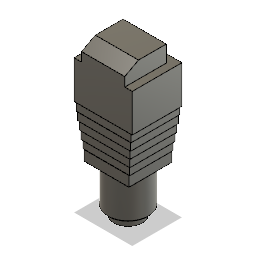
DIYbio orbital shaker bottom case (Autodesk Fusion 360 archive; units mm, degrees)
design "greenPlug"
Autodesk Fusion 360 part; units mm, degrees
sketch "Sketch1" plane through (0, 0, 0) normal (0, 1, 0) x (1, 0, 0)
  line L0 (5.245, -3.385) -> (-5.245, -3.385)
  line L1 (-5.245, -3.385) -> (-5.245, 3.385)
  line L2 (-5.245, 3.385) -> (5.245, 3.385)
  line L3 (5.245, 3.385) -> (5.245, -3.385)
  line L4 (5.245, -3.385) -> (-5.245, 3.385) construction
  line L5 (-5.245, -3.385) -> (5.245, 3.385) construction
  line L6 (5.245, -6.6889) -> (-5.245, -6.6889)
  line L7 (-5.245, -6.6889) -> (-5.245, -3.3689)
  line L8 (-5.245, -3.3689) -> (5.245, -3.3689)
  line L9 (5.245, -3.3689) -> (5.245, -6.6889)
  line L10 (5.245, -6.6889) -> (-5.245, -3.3689) construction
  line L11 (-5.245, -6.6889) -> (5.245, -3.3689) construction
  point P0 (0, -5.0289)
  dimension "d1" = 6.77
  dimension "d2" = 10.49
  dimension "d5" = 3.32
  dimension "d6" = 10.49
  constraint perpendicular L0 L1
  constraint parallel L0 L2
  constraint parallel L1 L3
  constraint horizontal L0
  constraint coincident L4 origin
  constraint coincident L5 origin
  constraint perpendicular L6 L7
  constraint parallel L6 L8
  constraint parallel L7 L9
  constraint horizontal L6
  constraint coincident L10 P0
  constraint coincident L11 P0
  measures "d1" distance of L0.end L1.end
  measures "d2" distance of L1.end L2.end
  measures "d5" distance of L6.end L7.end
  measures "d6" distance of L7.end L8.end
extrude "Extrude2" add sketch "Sketch1" along normal blind 3.99 contours L0 L6 L7 L9
extrude "Extrude1" add sketch "Sketch1" along normal blind 3.99 contours L0 L1 L3 L7 L8 L9 | L1 L2 L3 L8
sketch "Sketch2" plane through (-5.245, 0, 0) normal (-1, 0, 0) x (0, 0, 1)
  line L0 (-3.385, 0) -> (6.6889, 0)
  line L1 (6.6889, 0) -> (6.6889, 3.99)
  line L2 (6.6889, 3.99) -> (-3.385, 3.99)
  line L3 (-3.385, 3.99) -> (-3.385, 0)
  line L4 (6.6889, 3.99) -> (6.6889, 2.2)
  line L5 (6.6889, 3.99) -> (3.3689, 3.99)
  line L6 (3.3689, 3.99) -> (6.6889, 2.2)
  dimension "d9" = 1.79
  dimension "d10" = 3.32
  constraint coincident L1.end L2.start
  constraint perpendicular L2 L4
  constraint perpendicular L1 L5
  measures "d9" distance of L1.end L4.end
  measures "d10" distance of L1.end L5.end
extrude "Extrude3" cut sketch "Sketch2" against normal up to surface (10.49 mm away) contours L1 L2 L4 L5 L6
sketch "Sketch4" plane through (0, 0, 0) normal (0, -1, 0) x (1, 0, 0)
  line L0 (5.245, -3.385) -> (5.245, 6.6889)
  line L1 (5.245, 6.6889) -> (-5.245, 6.6889)
  line L2 (-5.245, 6.6889) -> (-5.245, -3.385)
  line L3 (-5.245, -3.385) -> (5.245, -3.385)
  line L4 (-7.055, 6.6889) -> (7.055, 6.6889)
  line L5 (7.055, 6.6889) -> (7.055, -5.3611)
  line L6 (7.055, -5.3611) -> (-7.055, -5.3611)
  line L7 (-7.055, -5.3611) -> (-7.055, 6.6889)
  line L8 (5.245, 3.3689) -> (5.245, 6.6889)
  dimension "d15" = 14.11
  dimension "d16" = 12.05
  dimension "d19" = 1.81
  constraint horizontal L4
  constraint vertical L5
  constraint horizontal L6
  constraint vertical L7
  measures "d15" distance of L4.start L4.end
  measures "d16" distance of L4.start L6.end
  measures "d19" distance of L5 L8
extrude "Extrude4" add sketch "Sketch4" 1 faces at (-1.7483, 0, -0.027) along normal blind 9.14 contours L0 L2 L3 L4 L5 L6 L7 L8
sketch "Sketch5" plane through (0, -9.14, 0) normal (0, -1, 0) x (1, 0, 0)
  line L0 (-7.055, -5.3611) -> (7.055, -5.3611)
  line L1 (7.055, -5.3611) -> (7.055, 6.6889)
  line L2 (7.055, 6.6889) -> (-7.055, 6.6889)
  line L3 (-7.055, 6.6889) -> (-7.055, -5.3611)
  line L4 (-6.61, 6.5539) -> (6.61, 6.5539)
  line L5 (6.61, 6.5539) -> (6.61, -5.2261)
  line L6 (6.61, -5.2261) -> (-6.61, -5.2261)
  line L7 (-6.61, -5.2261) -> (-6.61, 6.5539)
  dimension "d20" = 13.22
  dimension "d21" = 11.78
  dimension "d24" = 0.445
  dimension "d25" = 0.135
  constraint horizontal L4
  constraint vertical L5
  constraint horizontal L6
  constraint vertical L7
  measures "d20" distance of L4.start L4.end
  measures "d21" distance of L4.start L6.end
  measures "d24" distance of L3 L7
  measures "d25" distance of L2 L4
extrude "Extrude5" add sketch "Sketch5" along normal blind 1.92 contours L4 L5 L6 L7
sketch "Sketch6" plane through (0, -11.06, 0) normal (0, -1, 0) x (1, 0, 0)
  line L0 (-6.61, -5.2261) -> (6.61, -5.2261)
  line L1 (6.61, -5.2261) -> (6.61, 6.5539)
  line L2 (6.61, 6.5539) -> (-6.61, 6.5539)
  line L3 (-6.61, 6.5539) -> (-6.61, -5.2261)
  line L4 (6.415, -5.1311) -> (-6.415, -5.1311)
  line L5 (-6.415, -5.1311) -> (-6.415, 6.4589)
  line L6 (-6.415, 6.4589) -> (6.415, 6.4589)
  line L7 (6.415, 6.4589) -> (6.415, -5.1311)
  line L8 (6.415, -5.1311) -> (-6.415, 6.4589) construction
  line L9 (-6.415, -5.1311) -> (6.415, 6.4589) construction
  point P0 (0, 0.6639)
  dimension "d26" = 12.83
  dimension "d27" = 11.59
  dimension "d28" = 0.195
  dimension "d29" = 0.095
  constraint perpendicular L4 L5
  constraint parallel L4 L6
  constraint parallel L5 L7
  constraint horizontal L4
  constraint coincident L8 P0
  constraint coincident L9 P0
  measures "d26" distance of L5.end L6.end
  measures "d27" distance of L4.end L5.end
  measures "d28" distance of L1 L7
  measures "d29" distance of L0 L4
extrude "Extrude6" add sketch "Sketch6" along normal blind 1.92 contours L4 L5 L6 L7
sketch "Sketch7" plane through (0, -12.98, 0) normal (0, -1, 0) x (1, 0, 0)
  line L0 (6.415, 6.4589) -> (-6.415, 6.4589)
  line L1 (-6.415, 6.4589) -> (-6.415, -5.1311)
  line L2 (-6.415, -5.1311) -> (6.415, -5.1311)
  line L3 (6.415, -5.1311) -> (6.415, 6.4589)
  line L4 (6.12, -4.9711) -> (-6.12, -4.9711)
  line L5 (-6.12, -4.9711) -> (-6.12, 6.2989)
  line L6 (-6.12, 6.2989) -> (6.12, 6.2989)
  line L7 (6.12, 6.2989) -> (6.12, -4.9711)
  line L8 (6.12, -4.9711) -> (-6.12, 6.2989) construction
  line L9 (-6.12, -4.9711) -> (6.12, 6.2989) construction
  point P0 (0, 0.6639)
  dimension "d32" = 12.24
  dimension "d33" = 11.27
  dimension "d34" = 0.16
  dimension "d35" = 0.295
  constraint perpendicular L4 L5
  constraint parallel L4 L6
  constraint parallel L5 L7
  constraint horizontal L4
  constraint coincident L8 P0
  constraint coincident L9 P0
  measures "d32" distance of L5.end L6.end
  measures "d33" distance of L4.end L5.end
  measures "d34" distance of L2 L4
  measures "d35" distance of L3 L7
extrude "Extrude7" add sketch "Sketch7" along normal blind 1.92 contours L4 L5 L6 L7
sketch "Sketch8" plane through (0, -14.9, 0) normal (0, -1, 0) x (1, 0, 0)
  line L0 (6.12, 6.2989) -> (-6.12, 6.2989)
  line L1 (-6.12, 6.2989) -> (-6.12, -4.9711)
  line L2 (-6.12, -4.9711) -> (6.12, -4.9711)
  line L3 (6.12, -4.9711) -> (6.12, 6.2989)
  line L4 (5.92, -4.8161) -> (-5.92, -4.8161)
  line L5 (-5.92, -4.8161) -> (-5.92, 6.1439)
  line L6 (-5.92, 6.1439) -> (5.92, 6.1439)
  line L7 (5.92, 6.1439) -> (5.92, -4.8161)
  line L8 (5.92, -4.8161) -> (-5.92, 6.1439) construction
  line L9 (-5.92, -4.8161) -> (5.92, 6.1439) construction
  point P0 (0, 0.6639)
  dimension "d38" = 10.96
  dimension "d39" = 11.84
  dimension "d40" = 0.2
  dimension "d41" = 0.155
  constraint perpendicular L4 L5
  constraint parallel L4 L6
  constraint parallel L5 L7
  constraint horizontal L4
  constraint coincident L8 P0
  constraint coincident L9 P0
  measures "d38" distance of L4.end L5.end
  measures "d39" distance of L5.end L6.end
  measures "d40" distance of L1 L5
  measures "d41" distance of L2 L4
extrude "Extrude8" add sketch "Sketch8" along normal blind 1.92 contours L4 L5 L6 L7
sketch "Sketch9" plane through (0, -16.82, 0) normal (0, -1, 0) x (1, 0, 0)
  line L0 (5.92, 6.1439) -> (-5.92, 6.1439)
  line L1 (-5.92, 6.1439) -> (-5.92, -4.8161)
  line L2 (-5.92, -4.8161) -> (5.92, -4.8161)
  line L3 (5.92, -4.8161) -> (5.92, 6.1439)
  line L4 (5.66, -4.6211) -> (-5.66, -4.6211)
  line L5 (-5.66, -4.6211) -> (-5.66, 5.9489)
  line L6 (-5.66, 5.9489) -> (5.66, 5.9489)
  line L7 (5.66, 5.9489) -> (5.66, -4.6211)
  line L8 (5.66, -4.6211) -> (-5.66, 5.9489) construction
  line L9 (-5.66, -4.6211) -> (5.66, 5.9489) construction
  point P0 (0, 0.6639)
  dimension "d44" = 11.32
  dimension "d45" = 10.57
  dimension "d46" = 0.195
  dimension "d47" = 0.26
  constraint perpendicular L4 L5
  constraint parallel L4 L6
  constraint parallel L5 L7
  constraint horizontal L4
  constraint coincident L8 P0
  constraint coincident L9 P0
  measures "d44" distance of L5.end L6.end
  measures "d45" distance of L4.end L5.end
  measures "d46" distance of L0 L6
  measures "d47" distance of L3 L7
extrude "Extrude9" add sketch "Sketch9" along normal blind 1.92 contours L4 L5 L6 L7
sketch "Sketch10" plane through (0, -18.74, 0) normal (0, -1, 0) x (1, 0, 0)
  line L0 (5.66, 5.9489) -> (-5.66, 5.9489)
  line L1 (-5.66, 5.9489) -> (-5.66, -4.6211)
  line L2 (-5.66, -4.6211) -> (5.66, -4.6211)
  line L3 (5.66, -4.6211) -> (5.66, 5.9489)
  line L4 (5.45, -4.5361) -> (-5.45, -4.5361)
  line L5 (-5.45, -4.5361) -> (-5.45, 5.8739)
  line L6 (-5.45, 5.8739) -> (5.45, 5.8739)
  line L7 (5.45, 5.8739) -> (5.45, -4.5361)
  line L8 (5.45, -4.5361) -> (-5.45, 5.8739) construction
  line L9 (-5.45, -4.5361) -> (5.45, 5.8739) construction
  point P0 (0, 0.6689)
  dimension "d50" = 10.41
  dimension "d51" = 10.9
  dimension "d52" = 0.21
  dimension "d53" = 0.085
  constraint perpendicular L4 L5
  constraint parallel L4 L6
  constraint parallel L5 L7
  constraint horizontal L4
  constraint coincident L8 P0
  constraint coincident L9 P0
  measures "d50" distance of L4.end L5.end
  measures "d51" distance of L5.end L6.end
  measures "d52" distance of L1 L5
  measures "d53" distance of L2 L4
extrude "Extrude10" add sketch "Sketch10" along normal blind 2.54 contours L4 L5 L6 L7
sketch "Sketch11" plane through (0, -21.28, 0) normal (0, -1, 0) x (1, 0, 0)
  line L0 (5.45, 5.8739) -> (-5.45, 5.8739)
  line L1 (-5.45, 5.8739) -> (-5.45, -4.5361)
  line L2 (-5.45, -4.5361) -> (5.45, -4.5361)
  line L3 (5.45, -4.5361) -> (5.45, 5.8739)
  circle A0 centre (0.0234, 0.6708) radius 4.965
  circle A1 centre (0.0234, 0.6708) radius 2.805
  circle A2 centre (0.0234, 0.6708) radius 1
  dimension "d56" = 9.93
  dimension "d59" = 5.61
  dimension "d62" = 2
  constraint concentric A0 A1
  constraint concentric A0 A2
  measures "d56" diameter of A0
  measures "d59" diameter of A1
  measures "d62" diameter of A2
extrude "Extrude13" add sketch "Sketch11" along normal blind 9.05 contours A2
extrude "Extrude12" add sketch "Sketch11" along normal blind 9.05 contours A0
fillet "Fillet1" radius 1 1 edges at (-0.9089, -30.33, 0.3092)
sketch "Sketch12" plane through (0, -30.33, 0) normal (0, -1, 0) x (1, 0, 0)
  circle A0 centre (0.0234, 0.6708) radius 2.805
  circle A1 centre (0.0234, 0.6708) radius 4.965
  circle A2 centre (0.0234, 0.6708) radius 3.46
  dimension "d66" = 6.92
  constraint concentric A0 A2
  measures "d66" diameter of A2
extrude "Extrude14" add sketch "Sketch12" along normal blind 2.07 contours A2
fillet "Fillet2" radius 0.2 1 edges at (-4.6056, -30.33, -1.1246)
